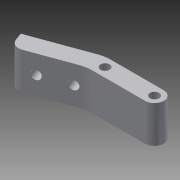
# Autodesk Inventor part: vrch
Saved by Autodesk Inventor 2014 (Build 180170000, 170)
## iProperties
Created: 2016-08-02
Part Number: vrch
Material: ABS plast
Document SubType Name: Modeling
Designer: Vojta3310
Mass: 2.79937 g
Surface Area: 18.617 cm^2
Volume: 2.64092 cm^3
Density: 1.06 g/cm^3
Appearance: Hladká – bílá
Author: Vojta3310
Autodesk Inventor part; units mm, degrees
ref_plane "YZ Plane" through (0, 0, 0) normal (1, 0, 0) x (0, 1, 0)
ref_plane "XZ Plane" through (0, 0, 0) normal (0, 1, 0) x (-1, 0, 0)
ref_plane "XY Plane" through (0, 0, 0) normal (0, 0, 1) x (1, 0, 0)
sketch "Náčrt2" plane through (-5.5, 0.074, 0) normal (0, 0, 1) x (1, 0, 0)
  line L0 (5.5, 7.926) -> (16.5, 7.926)
  circle A0 centre (13.5, 4.926) radius 1.5
  line L1 (16.5, 7.926) -> (16.5, 1.926)
  line L2 (16.5, 1.926) -> (-5.5, 1.926)
  line L3 (5.5, 7.926) -> (-5.5, 7.926)
  circle A1 centre (-2.5, 4.926) radius 1.5
  line L4 (-5.5, 7.926) -> (-5.5, 1.926)
  line L5 (-5.5, 7.926) -> (-25.5, 0.6466)
  line L6 (-5.5, 1.926) -> (-23.5716, -4.6515)
  line L7 (-23.5716, -4.6515) -> (-25.5, 0.6466)
  point P0 (5.5, -0.074)
  point P1 (5.5, -0.074)
  dimension "d2" = 3
  dimension "d5" = 3
  dimension "d4" = 8
  dimension "d3" = 5
  dimension "d1" = 3
  dimension "d0" = 3
  dimension "d11" = 3
  dimension "d22" = 20
  dimension "d23" = 20
  dimension "d39" = 3
  dimension "d40" = 22
  dimension "d41" = 3
  constraints: 16 end point, 2 centre point, 2 parallel, 2 perpendicular, 1 coincident, 1 collinear, 1 horizontal, 1 vertical
  measures "d2" diameter of A0
  measures "d5" distance from line of L0 A0.centre
  measures "d4" horizontal distance of point (5.5, -0.074) A0.centre
  measures "d3" vertical distance of A0.centre point (5.5, -0.074)
  measures "d1" distance from line of L1 A0.centre
  measures "d0" distance from line of A0.centre L2
  measures "d11" distance from line of L4 A1.centre
  measures "d22" angle of L3 L5
  measures "d23" horizontal distance of L3.end L5.end
  measures "d39" distance from line of L2 A1.centre
  measures "d40" distance of L1.end L2.end
  measures "d41" diameter of A1
extrude "Vysunutí1" add sketch "Náčrt2" along normal blind 12
fillet "Zaoblení2" radius 3 2 edges at (11, 2, 6) (11, 8, 6)
fillet "Zaoblení3" radius 10 2 edges at (-11, 2, 6) (-11, 8, 6)
fillet "Zaoblení4" radius 3 1 edges at (-29.0716, -4.5775, 6)
sketch "Náčrt3" plane through (-31, 0.7206, 12) normal (-0.3420201, 0.9396926, 0) x (0.9396926, 0.3420201, 0)
  line L0 (19.5203, 12) -> (0, 12) projected
  line L1 (0, 12) -> (0, 0) projected
  point P0 (28.884, 12)
  point P1 (16, 6)
  point P2 (6.5, 6)
  dimension "d27" = 6
  dimension "d28" = 6
  dimension "d29" = 9.5
  dimension "d30" = 16
  measures "d27" distance from line of L0 point (16, 6)
  measures "d28" distance from line of L0 point (6.5, 6)
  measures "d29" distance of point (6.5, 6) point (16, 6)
  measures "d30" distance from line of L1 point (16, 6)
hole "Díra2" at (-15.9649, 6.1929, 6) at (-24.892, 2.9437, 6) direction (0.3420201, -0.9396926, 0) diameter 2.9 end through all clearance for "Šroub se zápustnou hlavou ISO 2009/7046" size "M2.5" standard "ISO"
